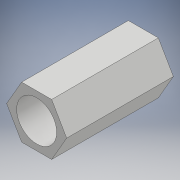
# Autodesk Inventor part: 7mmStandoff
Saved by Autodesk Inventor 2017 (Build 210142000, 142)
## iProperties
Created: 2019-03-15
Part Number: 7mmStandoff
Material: Generic
Document SubType Name: Modeling
Designer: Nicholas Cresswell
Density: 1 g/cm^3
Appearance: Default
Author: Nicholas Cresswell
Autodesk Inventor part; units mm, degrees
ref_plane "YZ Plane" through (0, 0, 0) normal (1, 0, 0) x (0, 1, 0)
ref_plane "XZ Plane" through (0, 0, 0) normal (0, 1, 0) x (-1, 0, 0)
ref_plane "XY Plane" through (0, 0, 0) normal (0, 0, 1) x (1, 0, 0)
sketch "Sketch1" plane through (0, 0, 0) normal (0, 1, 0) x (-1, 0, 0)
  circle A0 centre (0, 0) radius 1.5
  circle A1 centre (0, 0) radius 2.25 construction
  line L0 (2.25, 0) -> (1.125, -1.9486)
  line L1 (1.125, -1.9486) -> (-1.125, -1.9486)
  line L2 (-1.125, -1.9486) -> (-2.25, 0)
  line L3 (-2.25, 0) -> (-1.125, 1.9486)
  line L4 (-1.125, 1.9486) -> (1.125, 1.9486)
  line L5 (1.125, 1.9486) -> (2.25, 0)
  dimension "d1" = 4.5
  dimension "d0" = 3
  constraints: 12 end point, 3 coincident, 1 centre point, 1 horizontal alignment, 15 other
  measures "d0" diameter of A0
extrude "Extrusion1" add sketch "Sketch1" along normal blind 8
body "Solid1"
